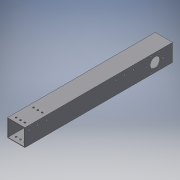
# Autodesk Inventor part: ATACHMENT BAR
Saved by Autodesk Inventor 2018.3 (Build 223284000, 284)
## iProperties
Created: 2019-01-26
Part Number: ATACHMENT BAR
Material: Generic
Document SubType Name: Modeling
Designer: s-4008082
Density: 1 g/cm^3
Appearance: Default
Author: s-4008082
Autodesk Inventor part; units mm, degrees
ref_plane "YZ Plane" through (0, 0, 0) normal (1, 0, 0) x (0, 1, 0)
ref_plane "XZ Plane" through (0, 0, 0) normal (0, 1, 0) x (-1, 0, 0)
ref_plane "XY Plane" through (0, 0, 0) normal (0, 0, 1) x (1, 0, 0)
sketch "Sketch1" plane through (0, 0, 0) normal (0, 0, 1) x (1, 0, 0)
  line L0 (0, 0) -> (-50.8, 0)
  line L1 (-50.8, 0) -> (-50.8, 50.8)
  line L2 (-50.8, 50.8) -> (0, 50.8)
  line L3 (0, 50.8) -> (0, 0)
  line L4 (-49.149, 49.149) -> (-1.651, 49.149)
  line L5 (-1.651, 49.149) -> (-1.651, 1.651)
  line L6 (-1.651, 1.651) -> (-49.149, 1.651)
  line L7 (-49.149, 1.651) -> (-49.149, 49.149)
  dimension "d0" = 50.8
  dimension "d1" = 50.8
  dimension "d2" = 1.651
  dimension "d3" = 1.651
  dimension "d4" = 1.651
  dimension "d5" = 1.651
  constraints: 16 end point, 4 parallel, 2 horizontal, 2 perpendicular
  measures "d0" distance of L0.end L1.end
  measures "d1" distance of L1.end L2.end
  measures "d2" distance between parallel lines of L1 L7
  measures "d3" distance between parallel lines of L2 L4
  measures "d4" distance between parallel lines of L3 L5
  measures "d5" distance between parallel lines of L0 L6
extrude "Extrusion1" add sketch "Sketch1" along normal blind 431.8
sketch "Sketch2" plane through (-50.8, 0, 0) normal (-1, 0, 0) x (0, 0, 1)
  circle A0 centre (114.3, 38.1) radius 2.5797
  circle A1 centre (139.7, 38.1) radius 2.5797
  circle A2 centre (165.1, 38.1) radius 2.5797
  circle A3 centre (368.3, 38.1) radius 2.5797
  circle A4 centre (393.7, 38.1) radius 2.5797
  circle A5 centre (419.1, 38.1) radius 2.5797
  line L0 (0, 0) -> (0, 50.8) projected
  line L1 (431.8, 50.8) -> (431.8, 0) projected
  line L2 (0, 50.8) -> (431.8, 50.8) projected
  dimension "d8" = 114.3
  dimension "d9" = 25.4
  dimension "d10" = 25.4
  dimension "d11" = 25.4
  dimension "d12" = 25.4
  dimension "d13" = 12.7
  dimension "d14" = 5.1594
  dimension "d15" = 5.1594
  dimension "d16" = 5.1594
  dimension "d19" = 5.1594
  dimension "d20" = 5.1594
  dimension "d21" = 5.1594
  dimension "d22" = 12.7
  dimension "d23" = 12.7
  dimension "d24" = 12.7
  dimension "d25" = 12.7
  dimension "d26" = 12.7
  dimension "d27" = 12.7
  constraints: 6 centre point
  measures "d8" distance from line of L0 A0.centre
  measures "d9" distance of A0.centre A1.centre
  measures "d10" distance of A1.centre A2.centre
  measures "d11" distance of A4.centre A3.centre
  measures "d12" distance of A4.centre A5.centre
  measures "d13" distance from line of L1 A5.centre
  measures "d14" diameter of A5
  measures "d15" diameter of A4
  measures "d16" diameter of A3
  measures "d19" diameter of A2
  measures "d20" diameter of A1
  measures "d21" diameter of A0
  measures "d22" distance from line of L2 A2.centre
  measures "d23" distance from line of L2 A1.centre
  measures "d24" distance from line of L2 A0.centre
  measures "d25" distance from line of L2 A3.centre
  measures "d26" distance from line of L2 A4.centre
  measures "d27" distance from line of L2 A5.centre
extrude "Extrusion2" cut sketch "Sketch2" against normal blind 279.4
sketch "Sketch5" plane through (0, 0, 0) normal (1, 0, 0) x (0, 0, -1)
  circle A0 centre (-50.8, 25.4) radius 9.525
  circle A1 centre (-26.9875, 25.4) radius 2.5797
  line L0 (0, 50.8) -> (0, 0) projected
  circle A2 centre (-50.8, 25.4) radius 23.8125 construction
  line L1 (0, 0) -> (-431.8, 0) projected
  circle A3 centre (-50.8, 25.4) radius 23.8125 construction
  circle A4 centre (-38.8938, 46.0222) radius 2.5797
  circle A5 centre (-50.8, 25.4) radius 23.8125 construction
  circle A6 centre (-62.7062, 46.0222) radius 2.5797
  circle A7 centre (-50.8, 25.4) radius 23.8125 construction
  circle A8 centre (-74.6125, 25.4) radius 2.5797
  circle A9 centre (-50.8, 25.4) radius 23.8125 construction
  circle A10 centre (-62.7063, 4.7778) radius 2.5797
  circle A11 centre (-50.8, 25.4) radius 23.8125 construction
  circle A12 centre (-38.8938, 4.7778) radius 2.5797
  dimension "d36" = 50.8
  dimension "d37" = 23.8125
  dimension "d38" = 19.05
  dimension "d39" = 5.1594
  dimension "d40" = 25.4
  dimension "d41" = 25.4
  dimension "d44" = 360
  constraints: 7 centre point, 3 coincident, 2 horizontal alignment, 39 other
  measures "d36" distance from line of L0 A0.centre
  measures "d37" distance of A0.centre A1.centre
  measures "d38" diameter of A0
  measures "d39" diameter of A1
  measures "d40" distance from line of L1 A1.centre
  measures "d41" distance from line of L1 A0.centre
extrude "Extrusion4" cut sketch "Sketch5" against normal blind 50.8 contours A1 | A4 | A6 | A8 | A10 | A12
sketch "Sketch6" plane through (0, 0, 0) normal (1, 0, 0) x (0, 0, -1)
  circle A0 centre (-50.8, 25.4) radius 14.605
  line L0 (0, 0) -> (-431.8, 0) projected
  circle A1 centre (-26.9875, 25.4) radius 2.5797 projected
  dimension "d48" = 25.4
  dimension "d49" = 23.8125
  dimension "d50" = 29.21
  constraints: 1 centre point
  measures "d48" distance from line of L0 A0.centre
  measures "d49" distance of A1.centre A0.centre
  measures "d50" diameter of A0
extrude "Extrusion5" cut sketch "Sketch6" against normal blind 50.8 contours A0
sketch "Sketch7" plane through (-50.8, 0, 0) normal (0, -1, 0) x (1, 0, 0)
  circle A0 centre (12.7, 419.1) radius 2.5797
  circle A1 centre (38.1, 419.1) radius 2.5797
  line L0 (49.149, 0) -> (49.149, 431.8) projected
  line L1 (0, 431.8) -> (50.8, 431.8) projected
  circle A2 centre (25.4, 419.1) radius 2.5797
  line L2 (50.8, 0) -> (50.8, 431.8) projected
  line L3 (38.1, 419.1) -> (38.1, 368.3) construction
  line L4 (38.1, 419.1) -> (88.9, 419.1) construction
  line L5 (25.4, 419.1) -> (25.4, 368.3) construction
  line L6 (12.7, 419.1) -> (12.7, 368.3) construction
  circle A3 centre (38.1, 368.3) radius 2.5797
  circle A4 centre (25.4, 368.3) radius 2.5797
  circle A5 centre (12.7, 368.3) radius 2.5797
  dimension "d53" = 5.1594
  dimension "d54" = 25.4
  dimension "d56" = 12.7
  dimension "d57" = 5.1594
  dimension "d58" = 5.1594
  dimension "d59" = 12.7
  dimension "d60" = 25.4
  dimension "d61" = 12.7
  dimension "d62" = 12.7
  dimension "d65" = 50.8
  dimension "d66" = 90
  dimension "d67" = 50.8
  dimension "d68" = 50.8
  dimension "d69" = 5.1594
  dimension "d70" = 5.1594
  dimension "d71" = 5.1594
  constraints: 8 end point, 6 centre point, 3 coincident, 3 vertical, 1 horizontal, 1 perpendicular
  measures "d53" diameter of A0
  measures "d54" distance of L6.start L3.start
  measures "d56" distance from line of L1 L3.start
  measures "d57" diameter of A2
  measures "d58" diameter of A1
  measures "d59" distance from line of L1 L6.start
  measures "d60" distance from line of L2 L5.start
  measures "d61" distance from line of L1 L5.start
  measures "d62" distance from line of L2 L3.start
  measures "d65" distance of L3.start L3.end
  measures "d66" angle of L3 L4
  measures "d67" distance of L5.start L5.end
  measures "d68" distance of L6.start L6.end
  measures "d69" diameter of A3
  measures "d70" diameter of A4
  measures "d71" diameter of A5
extrude "Extrusion7" cut sketch "Sketch7" against normal blind 127
equation "\"d3\" = d2"
equation "\"d4\" = d2"
equation "\"d5\" = d2"
equation "\"d10\" = d9"
equation "\"d11\" = d9"
equation "\"d15\" = d14"
equation "\"d16\" = d14"
equation "\"d19\" = d14"
equation "\"d20\" = d14"
equation "\"d21\" = d14"
equation "\"d26\" = d25"
equation "\"d27\" = d25"
equation "\"d57\" = d53"
equation "\"d58\" = d57"
body "Solid1"
